Autodesk Inventor part; units mm, degrees
note: some values were not read from the file. Chosen so that the rebuilt part matches the saved one: sketch regions of "Extrusion1".
(part 2 of 3)
  ellipse E482 centre (82.4896, 103.4568) end of major axis (81.6396, 103.4569) minor radius 0.8452 projected
  ellipse E483 centre (90.1098, 108.5077) end of major axis (89.3598, 108.5077) minor radius 0.7458 projected
  ellipse E484 centre (68.5696, 103.4576) end of major axis (66.5696, 103.4577) minor radius 1.9887 projected
  ellipse E485 centre (71.1098, 108.5087) end of major axis (70.3598, 108.5088) minor radius 0.7458 projected
  ellipse E486 centre (95.7978, 108.1793) end of major axis (95.5478, 108.1793) minor radius 0.2486 projected
  ellipse E487 centre (9.5448, 108.1839) end of major axis (9.2948, 108.1839) minor radius 0.2486 projected
  ellipse E488 centre (-152.6552, 108.1925) end of major axis (-152.9052, 108.1925) minor radius 0.2486 projected
  ellipse E489 centre (-102.1004, 103.4667) end of major axis (-102.9504, 103.4667) minor radius 0.8452 projected
  ellipse E490 centre (-112.2604, 103.4672) end of major axis (-113.1104, 103.4673) minor radius 0.8452 projected
  ellipse E491 centre (-104.6402, 108.5181) end of major axis (-105.3902, 108.5181) minor radius 0.7458 projected
  ellipse E492 centre (2.2348, 108.5124) end of major axis (1.4848, 108.5124) minor radius 0.7458 projected
  ellipse E493 centre (-5.3854, 103.4615) end of major axis (-6.2354, 103.4616) minor radius 0.8452 projected
  ellipse E494 centre (-0.3054, 103.4613) end of major axis (-2.3054, 103.4614) minor radius 1.9887 projected
  ellipse E495 centre (-29.1354, 103.4628) end of major axis (-29.9854, 103.4628) minor radius 0.8452 projected
  ellipse E496 centre (-27.8653, 105.9884) end of major axis (-28.6153, 105.9884) minor radius 0.7458 projected
  ellipse E497 centre (-21.5152, 108.5137) end of major axis (-22.2652, 108.5137) minor radius 0.7458 projected
  ellipse E498 centre (-59.6802, 108.1876) end of major axis (-61.0302, 108.1876) minor radius 1.3424 projected
  ellipse E499 centre (-61.112, 109.6114) end of major axis (-61.362, 109.6114) minor radius 0.2486 projected
  ellipse E500 centre (-58.2484, 106.7637) end of major axis (-58.4984, 106.7637) minor radius 0.2486 projected
  ellipse E501 centre (-58.2482, 109.6113) end of major axis (-58.4982, 109.6113) minor radius 0.2486 projected
  ellipse E502 centre (-59.6803, 106.174) end of major axis (-59.9303, 106.174) minor radius 0.2486 projected
  ellipse E503 centre (-57.6552, 108.1875) end of major axis (-57.9052, 108.1875) minor radius 0.2486 projected
  ellipse E504 centre (-59.6801, 110.2011) end of major axis (-59.9301, 110.2011) minor radius 0.2486 projected
  ellipse E505 centre (-50.03, 110.4243) end of major axis (-51.555, 110.4244) minor radius 1.5164 projected
  ellipse E506 centre (-61.7052, 108.1877) end of major axis (-61.9552, 108.1877) minor radius 0.2486 projected
  ellipse E507 centre (-187.7652, 108.5225) end of major axis (-188.5152, 108.5226) minor radius 0.7458 projected
  ellipse E508 centre (-156.1121, 106.7689) end of major axis (-156.3621, 106.7689) minor radius 0.2486 projected
  ellipse E509 centre (-154.6802, 108.1926) end of major axis (-156.0302, 108.1927) minor radius 1.3424 projected
  ellipse E510 centre (-153.2482, 109.6163) end of major axis (-153.4982, 109.6164) minor radius 0.2486 projected
  ellipse E511 centre (-156.112, 109.6165) end of major axis (-156.362, 109.6165) minor radius 0.2486 projected
  ellipse E512 centre (-156.7052, 108.1927) end of major axis (-156.9552, 108.1928) minor radius 0.2486 projected
  ellipse E513 centre (-154.6801, 110.2062) end of major axis (-154.9301, 110.2062) minor radius 0.2486 projected
  ellipse E514 centre (-164.33, 110.4304) end of major axis (-165.855, 110.4305) minor radius 1.5164 projected
  ellipse E515 centre (-190.3054, 103.4714) end of major axis (-192.3054, 103.4715) minor radius 1.9887 projected
  ellipse E516 centre (178.1668, 51.4973) end of major axis (177.9168, 51.4973) minor radius 0.2486 projected
  ellipse E517 centre (132.8568, 51.8278) end of major axis (132.1068, 51.8279) minor radius 0.7458 projected
  ellipse E518 centre (130.3176, 65.6692) end of major axis (128.3176, 65.6693) minor radius 1.9887 projected
  ellipse E519 centre (145.5077, 68.194) end of major axis (144.7577, 68.1941) minor radius 0.7458 projected
  ellipse E520 centre (168.3176, 65.6672) end of major axis (166.3176, 65.6673) minor radius 1.9887 projected
  ellipse E521 centre (149.3176, 65.6682) end of major axis (147.3176, 65.6683) minor radius 1.9887 projected
  ellipse E522 centre (173.3976, 65.6669) end of major axis (172.5476, 65.667) minor radius 0.8452 projected
  ellipse E523 centre (145.5087, 87.0866) end of major axis (144.7587, 87.0866) minor radius 0.7458 projected
  ellipse E524 centre (144.2386, 84.561) end of major axis (143.3886, 84.5611) minor radius 0.8452 projected
  ellipse E525 centre (149.3186, 84.5607) end of major axis (147.3186, 84.5608) minor radius 1.9887 projected
  ellipse E526 centre (168.3186, 84.5597) end of major axis (166.3186, 84.5598) minor radius 1.9887 projected
  ellipse E527 centre (163.2386, 84.56) end of major axis (162.3886, 84.56) minor radius 0.8452 projected
  ellipse E528 centre (139.8182, 77.1285) end of major axis (139.5682, 77.1285) minor radius 0.2486 projected
  ellipse E529 centre (138.3861, 73.6913) end of major axis (138.1361, 73.6913) minor radius 0.2486 projected
  ellipse E530 centre (138.3863, 76.5388) end of major axis (138.1363, 76.5389) minor radius 0.2486 projected
  ellipse E531 centre (141.25, 76.5387) end of major axis (141, 76.5387) minor radius 0.2486 projected
  ellipse E532 centre (139.8181, 75.115) end of major axis (138.4681, 75.115) minor radius 1.3424 projected
  ellipse E533 centre (141.8431, 75.1149) end of major axis (141.5931, 75.1149) minor radius 0.2486 projected
  ellipse E534 centre (135.3986, 84.5615) end of major axis (134.5486, 84.5615) minor radius 0.8452 projected
  ellipse E535 centre (139.818, 73.1014) end of major axis (139.568, 73.1014) minor radius 0.2486 projected
  ellipse E536 centre (126.5087, 87.0876) end of major axis (125.7587, 87.0876) minor radius 0.7458 projected
  ellipse E537 centre (125.2376, 65.6695) end of major axis (124.3876, 65.6695) minor radius 0.8452 projected
  ellipse E538 centre (126.5077, 68.1951) end of major axis (125.7577, 68.1951) minor radius 0.7458 projected
  ellipse E539 centre (63.4886, 84.5653) end of major axis (62.6386, 84.5654) minor radius 0.8452 projected
  ellipse E540 centre (73.6486, 84.5648) end of major axis (72.7986, 84.5648) minor radius 0.8452 projected
  ellipse E541 centre (113.8573, 61.2751) end of major axis (113.1073, 61.2751) minor radius 0.7458 projected
  ellipse E542 centre (118.3177, 68.0563) end of major axis (116.7927, 68.0564) minor radius 1.5164 projected
  ellipse E543 centre (-73.9314, 84.5727) end of major axis (-75.9314, 84.5728) minor radius 1.9887 projected
  ellipse E544 centre (-68.8514, 84.5724) end of major axis (-69.7014, 84.5724) minor radius 0.8452 projected
  ellipse E545 centre (-68.2423, 68.2055) end of major axis (-68.9923, 68.2055) minor radius 0.7458 projected
  ellipse E546 centre (-58.7413, 87.0975) end of major axis (-59.4913, 87.0975) minor radius 0.7458 projected
  ellipse E547 centre (-61.8922, 70.7307) end of major axis (-62.6422, 70.7308) minor radius 0.7458 projected
  ellipse E548 centre (-50.5124, 65.6789) end of major axis (-51.3624, 65.6789) minor radius 0.8452 projected
  ellipse E549 centre (-69.5124, 65.6799) end of major axis (-70.3624, 65.6799) minor radius 0.8452 projected
  ellipse E550 centre (-49.2423, 68.2044) end of major axis (-49.9923, 68.2045) minor radius 0.7458 projected
  ellipse E551 centre (-21.3524, 65.6773) end of major axis (-22.2024, 65.6774) minor radius 0.8452 projected
  ellipse E552 centre (-26.4324, 65.6776) end of major axis (-28.4324, 65.6777) minor radius 1.9887 projected
  ellipse E553 centre (-26.4319, 75.7264) end of major axis (-27.7819, 75.7265) minor radius 1.3424 projected
  ellipse E554 centre (-27.8639, 74.3027) end of major axis (-28.1139, 74.3027) minor radius 0.2486 projected
  ellipse E555 centre (-35.9314, 84.5706) end of major axis (-37.9314, 84.5707) minor radius 1.9887 projected
  ellipse E556 centre (-20.7413, 87.0954) end of major axis (-21.4913, 87.0955) minor radius 0.7458 projected
  ellipse E557 centre (-40.3524, 65.6783) end of major axis (-41.2024, 65.6784) minor radius 0.8452 projected
  ellipse E558 centre (-39.7413, 87.0965) end of major axis (-40.4913, 87.0965) minor radius 0.7458 projected
  ellipse E559 centre (-42.8922, 70.7297) end of major axis (-43.6422, 70.7298) minor radius 0.7458 projected
  ellipse E560 centre (-45.4324, 65.6786) end of major axis (-47.4324, 65.6787) minor radius 1.9887 projected
  ellipse E561 centre (13.9436, 84.568) end of major axis (11.9436, 84.5681) minor radius 1.9887 projected
  ellipse E562 centre (10.1337, 87.0938) end of major axis (9.3837, 87.0938) minor radius 0.7458 projected
  ellipse E563 centre (2.0431, 76.3752) end of major axis (0.0431, 76.3753) minor radius 1.9887 projected
  ellipse E564 centre (-16.9314, 84.5696) end of major axis (-18.9314, 84.5697) minor radius 1.9887 projected
  ellipse E565 centre (-2.3524, 65.6763) end of major axis (-3.2024, 65.6763) minor radius 0.8452 projected
  ellipse E566 centre (31.9998, 71.8214) end of major axis (31.7498, 71.8214) minor radius 0.2486 projected
  ellipse E567 centre (25.8431, 76.3739) end of major axis (23.8431, 76.374) minor radius 1.9887 projected
  ellipse E568 centre (31.9996, 68.9738) end of major axis (31.7496, 68.9738) minor radius 0.2486 projected
  ellipse E569 centre (30.5678, 70.3977) end of major axis (29.2178, 70.3977) minor radius 1.3424 projected
  ellipse E570 centre (28.5428, 70.3978) end of major axis (28.2928, 70.3978) minor radius 0.2486 projected
  ellipse E571 centre (18.6926, 65.6752) end of major axis (16.6926, 65.6753) minor radius 1.9887 projected
  ellipse E572 centre (21.2328, 70.7263) end of major axis (20.4828, 70.7263) minor radius 0.7458 projected
  ellipse E573 centre (-0.1432, 51.8349) end of major axis (-0.8932, 51.835) minor radius 0.7458 projected
  ellipse E574 centre (-57.1432, 51.838) end of major axis (-57.8932, 51.838) minor radius 0.7458 projected
  ellipse E575 centre (-76.1432, 51.839) end of major axis (-76.8932, 51.839) minor radius 0.7458 projected
  ellipse E576 centre (23.6068, 51.8336) end of major axis (22.8568, 51.8337) minor radius 0.7458 projected
  ellipse E577 centre (32.5928, 70.3976) end of major axis (32.3428, 70.3976) minor radius 0.2486 projected
  ellipse E578 centre (-109.907, 74.4681) end of major axis (-110.157, 74.4681) minor radius 0.2486 projected
  ellipse E579 centre (-102.4324, 65.6816) end of major axis (-104.4324, 65.6817) minor radius 1.9887 projected
  ellipse E580 centre (-78.3524, 65.6804) end of major axis (-79.2024, 65.6804) minor radius 0.8452 projected
  ellipse E581 centre (-88.5124, 65.6809) end of major axis (-89.3624, 65.6809) minor radius 0.8452 projected
  ellipse E582 centre (-87.2423, 68.2065) end of major axis (-87.9923, 68.2065) minor radius 0.7458 projected
  ellipse E583 centre (-96.7413, 87.0995) end of major axis (-97.4913, 87.0995) minor radius 0.7458 projected
  ellipse E584 centre (-110.5002, 73.0443) end of major axis (-110.7502, 73.0443) minor radius 0.2486 projected
  ellipse E585 centre (-191.7413, 87.1046) end of major axis (-192.4913, 87.1046) minor radius 0.7458 projected
  ellipse E586 centre (-187.9314, 84.5787) end of major axis (-189.9314, 84.5788) minor radius 1.9887 projected
  ellipse E587 centre (-174.0114, 84.578) end of major axis (-174.8614, 84.578) minor radius 0.8452 projected
  ellipse E588 centre (-172.7413, 87.1036) end of major axis (-173.4913, 87.1036) minor radius 0.7458 projected
  ellipse E589 centre (-153.7413, 87.1025) end of major axis (-154.4913, 87.1026) minor radius 0.7458 projected
  ellipse E590 centre (-163.8514, 84.5775) end of major axis (-164.7014, 84.5775) minor radius 0.8452 projected
  ellipse E591 centre (-113.3638, 75.892) end of major axis (-113.6138, 75.8921) minor radius 0.2486 projected
  ellipse E592 centre (-111.932, 74.4682) end of major axis (-113.282, 74.4682) minor radius 1.3424 projected
  ellipse E593 centre (-110.5, 75.8919) end of major axis (-110.75, 75.8919) minor radius 0.2486 projected
  ellipse E594 centre (-113.957, 74.4683) end of major axis (-114.207, 74.4683) minor radius 0.2486 projected
  ellipse E595 centre (-117.0114, 84.575) end of major axis (-117.8614, 84.575) minor radius 0.8452 projected
  ellipse E596 centre (-115.7413, 87.1005) end of major axis (-116.4913, 87.1006) minor radius 0.7458 projected
  ellipse E597 centre (-130.9314, 84.5757) end of major axis (-132.9314, 84.5758) minor radius 1.9887 projected
  ellipse E598 centre (-149.9314, 84.5767) end of major axis (-151.9314, 84.5768) minor radius 1.9887 projected
  ellipse E599 centre (-182.2423, 68.2115) end of major axis (-182.9923, 68.2116) minor radius 0.7458 projected
  ellipse E600 centre (-183.5124, 65.686) end of major axis (-184.3624, 65.686) minor radius 0.8452 projected
  ellipse E601 centre (-178.4324, 65.6857) end of major axis (-180.4324, 65.6858) minor radius 1.9887 projected
  ellipse E602 centre (-163.2423, 68.2105) end of major axis (-163.9923, 68.2106) minor radius 0.7458 projected
  ellipse E603 centre (-137.8922, 70.7348) end of major axis (-138.6422, 70.7348) minor radius 0.7458 projected
  ellipse E604 centre (-144.2423, 68.2095) end of major axis (-144.9923, 68.2095) minor radius 0.7458 projected
  ellipse E605 centre (-140.4324, 65.6837) end of major axis (-142.4324, 65.6838) minor radius 1.9887 projected
  ellipse E606 centre (-126.5124, 65.6829) end of major axis (-127.3624, 65.683) minor radius 0.8452 projected
  ellipse E607 centre (-135.3524, 65.6834) end of major axis (-136.2024, 65.6834) minor radius 0.8452 projected
  ellipse E608 centre (-111.9321, 72.4546) end of major axis (-112.1821, 72.4546) minor radius 0.2486 projected
  ellipse E609 centre (-118.8922, 70.7338) end of major axis (-119.6422, 70.7338) minor radius 0.7458 projected
  ellipse E610 centre (-192.3524, 65.6864) end of major axis (-193.2024, 65.6865) minor radius 0.8452 projected
  ellipse E611 centre (-133.1432, 51.842) end of major axis (-133.8932, 51.8421) minor radius 0.7458 projected
  ellipse E612 centre (-171.1432, 51.844) end of major axis (-171.8932, 51.8441) minor radius 0.7458 projected
  ellipse E613 centre (107.5092, 96.5349) end of major axis (106.7592, 96.5349) minor radius 0.7458 projected
  ellipse E614 centre (-14.3912, 89.6207) end of major axis (-15.1412, 89.6208) minor radius 0.7458 projected
  ellipse E615 centre (25.8439, 91.5277) end of major axis (24.3189, 91.5278) minor radius 1.5164 projected
  ellipse E616 centre (132.8588, 89.6129) end of major axis (132.1088, 89.6129) minor radius 0.7458 projected
  ellipse E617 centre (116.3991, 94.0088) end of major axis (115.5491, 94.0088) minor radius 0.8452 projected
  ellipse E618 centre (-90.3912, 89.6248) end of major axis (-91.1412, 89.6248) minor radius 0.7458 projected
  ellipse E619 centre (-71.3912, 89.6238) end of major axis (-72.1412, 89.6238) minor radius 0.7458 projected
  ellipse E620 centre (-164.3309, 95.2766) end of major axis (-166.3309, 95.2767) minor radius 1.9887 projected
  ellipse E621 centre (-166.3912, 89.6289) end of major axis (-167.1412, 89.6289) minor radius 0.7458 projected
  ellipse E622 centre (181.6238, 52.9209) end of major axis (181.3738, 52.9209) minor radius 0.2486 projected
  ellipse E623 centre (178.76, 52.921) end of major axis (178.51, 52.921) minor radius 0.2486 projected
  ellipse E624 centre (180.1919, 53.5107) end of major axis (179.9419, 53.5107) minor radius 0.2486 projected
  ellipse E625 centre (178.757, -3.7566) end of major axis (178.507, -3.7566) minor radius 0.2486 projected
  ellipse E626 centre (73.8545, 8.9399) end of major axis (73.4545, 8.94) minor radius 0.3977 projected
  ellipse E627 centre (81.4745, 8.9395) end of major axis (81.0745, 8.9396) minor radius 0.3977 projected
  ellipse E628 centre (125.2366, 46.777) end of major axis (124.3866, 46.777) minor radius 0.8452 projected
  ellipse E629 centre (126.5057, 30.41) end of major axis (125.7557, 30.41) minor radius 0.7458 projected
  ellipse E630 centre (135.3966, 46.7764) end of major axis (134.5466, 46.7765) minor radius 0.8452 projected
  ellipse E631 centre (137.791, 37.33) end of major axis (137.541, 37.33) minor radius 0.2486 projected
  ellipse E632 centre (154.3966, 46.7754) end of major axis (153.5466, 46.7754) minor radius 0.8452 projected
  ellipse E633 centre (141.841, 37.3298) end of major axis (141.591, 37.3298) minor radius 0.2486 projected
  ellipse E634 centre (138.3841, 35.9062) end of major axis (138.1341, 35.9062) minor radius 0.2486 projected
  ellipse E635 centre (139.816, 37.3299) end of major axis (138.466, 37.33) minor radius 1.3424 projected
  ellipse E636 centre (141.248, 38.7536) end of major axis (140.998, 38.7536) minor radius 0.2486 projected
  ellipse E637 centre (151.8558, 32.9343) end of major axis (151.1058, 32.9343) minor radius 0.7458 projected
  ellipse E638 centre (139.8159, 35.3164) end of major axis (139.5659, 35.3164) minor radius 0.2486 projected
  ellipse E639 centre (149.3155, 27.8831) end of major axis (147.3155, 27.8832) minor radius 1.9887 projected
  ellipse E640 centre (125.2355, 27.8844) end of major axis (124.3855, 27.8845) minor radius 0.8452 projected
  ellipse E641 centre (135.3955, 27.8839) end of major axis (134.5455, 27.8839) minor radius 0.8452 projected
  ellipse E642 centre (106.2355, 27.8854) end of major axis (105.3855, 27.8855) minor radius 0.8452 projected
  ellipse E643 centre (168.3155, 27.8821) end of major axis (166.3155, 27.8822) minor radius 1.9887 projected
  ellipse E644 centre (173.3966, 46.7744) end of major axis (172.5466, 46.7744) minor radius 0.8452 projected
  ellipse E645 centre (103.0764, 44.3917) end of major axis (101.0764, 44.3918) minor radius 1.9887 projected
  ellipse E646 centre (76.041, 37.3333) end of major axis (75.791, 37.3333) minor radius 0.2486 projected
  ellipse E647 centre (44.4866, 46.7813) end of major axis (43.6366, 46.7813) minor radius 0.8452 projected
  ellipse E648 centre (45.7557, 30.4143) end of major axis (45.0057, 30.4143) minor radius 0.7458 projected
  ellipse E649 centre (71.3145, 8.9401) end of major axis (70.9145, 8.9401) minor radius 0.3977 projected
  ellipse E650 centre (66.2345, 8.9403) end of major axis (65.8345, 8.9404) minor radius 0.3977 projected
  ellipse E651 centre (56.0745, 8.9409) end of major axis (55.6745, 8.9409) minor radius 0.3977 projected
  ellipse E652 centre (52.351, -1.1614) end of major axis (51.851, -1.1614) minor radius 0.4972 projected
  ellipse E653 centre (-9.6457, 4.6041) end of major axis (-10.3957, 4.6041) minor radius 0.7458 projected
  ellipse E654 centre (9.9939, -3.3318) end of major axis (9.5939, -3.3318) minor radius 0.3977 projected
  ellipse E655 centre (36.257, -3.749) end of major axis (36.007, -3.749) minor radius 0.2486 projected
  ellipse E656 centre (7.1662, 39.6986) end of major axis (6.9162, 39.6986) minor radius 0.2486 projected
  ellipse E657 centre (28.3558, 32.9409) end of major axis (27.6058, 32.9409) minor radius 0.7458 projected
  ellipse E658 centre (26.1466, 46.7822) end of major axis (25.2966, 46.7823) minor radius 0.8452 projected
  ellipse E659 centre (126.5067, 49.3025) end of major axis (125.7567, 49.3026) minor radius 0.7458 projected
  ellipse E660 centre (-72.9958, 2.0818) end of major axis (-73.7458, 2.0819) minor radius 0.7458 projected
  ellipse E661 centre (-69.1838, 40.1103) end of major axis (-69.4338, 40.1103) minor radius 0.2486 projected
  ellipse E662 centre (-69.184, 36.0832) end of major axis (-69.434, 36.0832) minor radius 0.2486 projected
  ellipse E663 centre (-67.7521, 36.6729) end of major axis (-68.0021, 36.6729) minor radius 0.2486 projected
  ellipse E664 centre (-69.1839, 38.0968) end of major axis (-70.5339, 38.0968) minor radius 1.3424 projected
  ellipse E665 centre (-50.1845, 27.8938) end of major axis (-52.1845, 27.8939) minor radius 1.9887 projected
  ellipse E666 centre (-36.266, -0.4458) end of major axis (-37.116, -0.4457) minor radius 0.8452 projected
  ellipse E667 centre (-34.9958, 2.0798) end of major axis (-35.7458, 2.0798) minor radius 0.7458 projected
  ellipse E668 centre (-66.6457, 4.6071) end of major axis (-67.3957, 4.6072) minor radius 0.7458 projected
  ellipse E669 centre (-69.186, -0.444) end of major axis (-71.186, -0.4439) minor radius 1.9887 projected
  ellipse E670 centre (-54.6034, 46.7866) end of major axis (-55.4534, 46.7866) minor radius 0.8452 projected
  ellipse E671 centre (-40.6834, 46.7858) end of major axis (-42.6834, 46.7859) minor radius 1.9887 projected
  ellipse E672 centre (-45.7634, 46.7861) end of major axis (-46.6134, 46.7861) minor radius 0.8452 projected
  ellipse E673 centre (-35.6034, 46.7855) end of major axis (-36.4534, 46.7856) minor radius 0.8452 projected
  ellipse E674 centre (-64.7634, 46.7871) end of major axis (-65.6134, 46.7871) minor radius 0.8452 projected
  ellipse E675 centre (-26.106, -0.4463) end of major axis (-26.956, -0.4463) minor radius 0.8452 projected
  ellipse E676 centre (-26.1045, 27.8925) end of major axis (-26.9545, 27.8925) minor radius 0.8452 projected
  ellipse E677 centre (17.2567, 49.3084) end of major axis (16.5067, 49.3084) minor radius 0.7458 projected
  ellipse E678 centre (15.9866, 46.7828) end of major axis (15.1366, 46.7828) minor radius 0.8452 projected
  ellipse E679 centre (10.6231, 41.1222) end of major axis (10.3731, 41.1222) minor radius 0.2486 projected
  ellipse E680 centre (11.8955, 27.8905) end of major axis (11.0455, 27.8905) minor radius 0.8452 projected
  ellipse E681 centre (7.7592, 38.2747) end of major axis (7.5092, 38.2747) minor radius 0.2486 projected
  ellipse E682 centre (6.8155, 27.8907) end of major axis (4.8155, 27.8909) minor radius 1.9887 projected
  ellipse E683 centre (-16.6034, 46.7845) end of major axis (-17.4534, 46.7846) minor radius 0.8452 projected
  ellipse E684 centre (-7.1045, 27.8915) end of major axis (-7.9545, 27.8915) minor radius 0.8452 projected
  ellipse E685 centre (-17.266, -0.4468) end of major axis (-18.116, -0.4467) minor radius 0.8452 projected
  ellipse E686 centre (-15.9958, 2.0788) end of major axis (-16.7458, 2.0788) minor radius 0.7458 projected
  ellipse E687 centre (64.7567, 49.3058) end of major axis (64.0067, 49.3059) minor radius 0.7458 projected
  ellipse E688 centre (64.7557, 30.4133) end of major axis (64.0057, 30.4133) minor radius 0.7458 projected
  ellipse E689 centre (52.3513, 3.8898) end of major axis (51.8513, 3.8899) minor radius 0.4972 projected
  ellipse E690 centre (61.1545, 8.9406) end of major axis (60.7545, 8.9406) minor radius 0.3977 projected
  ellipse E691 centre (44.9851, 0.2062) end of major axis (44.6101, 0.2062) minor radius 0.3729 projected
  ellipse E692 centre (-148.9943, 30.4247) end of major axis (-149.7443, 30.4247) minor radius 0.7458 projected
  ellipse E693 centre (-129.9943, 30.4237) end of major axis (-130.7443, 30.4237) minor radius 0.7458 projected
  ellipse E694 centre (-140.1045, 27.8986) end of major axis (-140.9545, 27.8986) minor radius 0.8452 projected
  ellipse E695 centre (-131.2645, 27.8981) end of major axis (-132.1145, 27.8982) minor radius 0.8452 projected
  ellipse E696 centre (-95.1457, 4.6087) end of major axis (-95.8957, 4.6087) minor radius 0.7458 projected
  ellipse E697 centre (-112.2645, 27.8971) end of major axis (-113.1145, 27.8971) minor radius 0.8452 projected
  ellipse E698 centre (-107.1845, 27.8968) end of major axis (-109.1845, 27.8969) minor radius 1.9887 projected
  ellipse E699 centre (-92.606, -0.4427) end of major axis (-93.456, -0.4427) minor radius 0.8452 projected
  ellipse E700 centre (-102.766, -0.4422) end of major axis (-103.616, -0.4422) minor radius 0.8452 projected
  ellipse E701 centre (-97.686, -0.4425) end of major axis (-99.686, -0.4424) minor radius 1.9887 projected
  ellipse E702 centre (-139.4958, 2.0854) end of major axis (-140.2458, 2.0854) minor radius 0.7458 projected
  ellipse E703 centre (-149.6034, 46.7916) end of major axis (-150.4534, 46.7917) minor radius 0.8452 projected
  ellipse E704 centre (-92.6034, 46.7886) end of major axis (-93.4534, 46.7886) minor radius 0.8452 projected
  ellipse E705 centre (-139.4933, 49.3167) end of major axis (-140.2433, 49.3168) minor radius 0.7458 projected
  ellipse E706 centre (-82.4933, 49.3137) end of major axis (-83.2433, 49.3137) minor radius 0.7458 projected
  ellipse E707 centre (-83.4361, -3.1528) end of major axis (-83.6861, -3.1528) minor radius 0.2486 projected
  ellipse E708 centre (-168.9361, -3.1483) end of major axis (-169.1861, -3.1482) minor radius 0.2486 projected
  ellipse E709 centre (-169.2645, 27.9001) end of major axis (-170.1145, 27.9002) minor radius 0.8452 projected
  ellipse E710 centre (-159.7634, 46.7922) end of major axis (-160.6134, 46.7922) minor radius 0.8452 projected
  ellipse E711 centre (-159.1045, 27.8996) end of major axis (-159.9545, 27.8996) minor radius 0.8452 projected
  ellipse E712 centre (-152.1457, 4.6117) end of major axis (-152.8957, 4.6117) minor radius 0.7458 projected
  ellipse E713 centre (-187.6034, 46.7937) end of major axis (-188.4534, 46.7937) minor radius 0.8452 projected
  ellipse E714 centre (-170.368, -3.7379) end of major axis (-170.618, -3.7379) minor radius 0.2486 projected
  ellipse E715 centre (-180.6457, 4.6132) end of major axis (-181.3957, 4.6133) minor radius 0.7458 projected
  ellipse E716 centre (-177.4933, 49.3188) end of major axis (-178.2433, 49.3188) minor radius 0.7458 projected
  ellipse E717 centre (178.7598, 50.0734) end of major axis (178.5098, 50.0735) minor radius 0.2486 projected
  ellipse E718 centre (181.6207, -3.7567) end of major axis (181.3707, -3.7567) minor radius 0.2486 projected
  ellipse E719 centre (180.1889, -3.1669) end of major axis (179.9389, -3.1669) minor radius 0.2486 projected
  ellipse E720 centre (181.6236, 50.0733) end of major axis (181.3736, 50.0733) minor radius 0.2486 projected
  ellipse E721 centre (180.1918, 51.4972) end of major axis (178.8418, 51.4972) minor radius 1.3424 projected
  ellipse E722 centre (180.1917, 49.4836) end of major axis (179.9417, 49.4836) minor radius 0.2486 projected
  ellipse E723 centre (-211.5152, 108.5238) end of major axis (-212.2652, 108.5238) minor radius 0.7458 projected
  ellipse E724 centre (-202.1811, 91.6642) end of major axis (-203.5311, 91.6643) minor radius 1.3424 projected
  ellipse E725 centre (-204.2061, 91.6643) end of major axis (-204.4561, 91.6643) minor radius 0.2486 projected
  ellipse E726 centre (-201.2423, 68.2126) end of major axis (-201.9923, 68.2126) minor radius 0.7458 projected
  ellipse E727 centre (-209.1432, 51.8461) end of major axis (-209.8932, 51.8461) minor radius 0.7458 projected
  ellipse E728 centre (-205.9958, 2.0889) end of major axis (-206.7458, 2.089) minor radius 0.7458 projected
  ellipse E729 centre (180.1887, -7.194) end of major axis (179.9387, -7.194) minor radius 0.2486 projected
  ellipse E730 centre (178.7568, -6.6042) end of major axis (178.5068, -6.6041) minor radius 0.2486 projected
  ellipse E731 centre (178.1638, -5.1803) end of major axis (177.9138, -5.1803) minor radius 0.2486 projected
  ellipse E732 centre (181.6206, -6.6043) end of major axis (181.3706, -6.6043) minor radius 0.2486 projected
  ellipse E733 centre (180.1888, -5.1804) end of major axis (178.8388, -5.1804) minor radius 1.3424 projected
  ellipse E734 centre (182.2198, 108.1746) end of major axis (181.9698, 108.1747) minor radius 0.2486 projected
  ellipse E735 centre (182.2168, 51.497) end of major axis (181.9668, 51.4971) minor radius 0.2486 projected
  ellipse E736 centre (182.2138, -5.1806) end of major axis (181.9638, -5.1805) minor radius 0.2486 projected
  ellipse E737 centre (-252.0552, 108.1978) end of major axis (-253.4052, 108.1979) minor radius 1.3424 projected
  ellipse E738 centre (-250.6234, 106.774) end of major axis (-250.8734, 106.774) minor radius 0.2486 projected
  ellipse E739 centre (-253.4871, 106.7741) end of major axis (-253.7371, 106.7741) minor radius 0.2486 projected
  ellipse E740 centre (-250.6232, 109.6215) end of major axis (-250.8732, 109.6216) minor radius 0.2486 projected
  ellipse E741 centre (-253.487, 109.6217) end of major axis (-253.737, 109.6217) minor radius 0.2486 projected
  ellipse E742 centre (-252.0553, 106.1843) end of major axis (-252.3053, 106.1843) minor radius 0.2486 projected
  ellipse E743 centre (-250.6262, 52.9439) end of major axis (-250.8762, 52.944) minor radius 0.2486 projected
  ellipse E744 centre (-252.0582, 51.5202) end of major axis (-253.4082, 51.5203) minor radius 1.3424 projected
  ellipse E745 centre (-250.6264, 50.0964) end of major axis (-250.8764, 50.0964) minor radius 0.2486 projected
  ellipse E746 centre (-253.4902, 50.0965) end of major axis (-253.7402, 50.0965) minor radius 0.2486 projected
  ellipse E747 centre (-253.49, 52.9441) end of major axis (-253.74, 52.9441) minor radius 0.2486 projected
  ellipse E748 centre (-252.0581, 53.5338) end of major axis (-252.3081, 53.5338) minor radius 0.2486 projected
  ellipse E749 centre (-253.4932, -6.5811) end of major axis (-253.7432, -6.5811) minor radius 0.2486 projected
  ellipse E750 centre (-252.0612, -5.1574) end of major axis (-253.4112, -5.1573) minor radius 1.3424 projected
  ellipse E751 centre (-250.6294, -6.5812) end of major axis (-250.8794, -6.5812) minor radius 0.2486 projected
  ellipse E752 centre (-253.493, -3.7335) end of major axis (-253.743, -3.7335) minor radius 0.2486 projected
  ellipse E753 centre (-250.6293, -3.7337) end of major axis (-250.8793, -3.7336) minor radius 0.2486 projected
  ellipse E754 centre (-252.0611, -3.1438) end of major axis (-252.3111, -3.1438) minor radius 0.2486 projected
  ellipse E755 centre (-252.0583, 49.5067) end of major axis (-252.3083, 49.5067) minor radius 0.2486 projected
  ellipse E756 centre (-240.5134, 46.7965) end of major axis (-241.3634, 46.7965) minor radius 0.8452 projected
  ellipse E757 centre (-239.2433, 49.322) end of major axis (-239.9933, 49.3221) minor radius 0.7458 projected
  ellipse E758 centre (-250.0332, 51.5201) end of major axis (-250.2832, 51.5201) minor radius 0.2486 projected
  ellipse E759 centre (-242.5841, 34.8645) end of major axis (-244.1091, 34.8645) minor radius 1.5164 projected
  ellipse E760 centre (-242.8854, 103.4742) end of major axis (-243.7354, 103.4743) minor radius 0.8452 projected
  ellipse E761 centre (-240.2071, 72.6494) end of major axis (-241.7321, 72.6495) minor radius 1.5164 projected
  ellipse E762 centre (-242.5849, 19.7107) end of major axis (-244.5849, 19.7108) minor radius 1.9887 projected
  ellipse E763 centre (-250.0362, -5.1575) end of major axis (-250.2862, -5.1575) minor radius 0.2486 projected
  ellipse E764 centre (-240.186, -0.4349) end of major axis (-242.186, -0.4348) minor radius 1.9887 projected
  ellipse E765 centre (-243.9958, 2.091) end of major axis (-244.7458, 2.091) minor radius 0.7458 projected
  ellipse E766 centre (-245.266, -0.4346) end of major axis (-246.116, -0.4346) minor radius 0.8452 projected
  ellipse E767 centre (-250.0302, 108.1977) end of major axis (-250.2802, 108.1977) minor radius 0.2486 projected
  ellipse E768 centre (-224.9906, 41.1347) end of major axis (-225.2406, 41.1348) minor radius 0.2486 projected
  ellipse E769 centre (-223.5588, 39.7109) end of major axis (-224.9088, 39.7109) minor radius 1.3424 projected
  ellipse E770 centre (-222.127, 38.287) end of major axis (-222.377, 38.287) minor radius 0.2486 projected
  ellipse E771 centre (-224.9908, 38.2872) end of major axis (-225.2408, 38.2872) minor radius 0.2486 projected
  ellipse E772 centre (-222.1269, 41.1346) end of major axis (-222.3769, 41.1346) minor radius 0.2486 projected
  ellipse E773 centre (-225.5838, 39.711) end of major axis (-225.8338, 39.711) minor radius 0.2486 projected
  ellipse E774 centre (-223.5589, 37.6973) end of major axis (-223.8089, 37.6973) minor radius 0.2486 projected
  ellipse E775 centre (-235.7645, 27.9037) end of major axis (-236.6145, 27.9037) minor radius 0.8452 projected
  ellipse E776 centre (-234.4943, 30.4293) end of major axis (-235.2443, 30.4293) minor radius 0.7458 projected
  ellipse E777 centre (-228.1442, 32.9546) end of major axis (-228.8942, 32.9546) minor radius 0.7458 projected
  ellipse E778 centre (-230.6845, 27.9034) end of major axis (-232.6845, 27.9035) minor radius 1.9887 projected
  ellipse E779 centre (-225.6045, 27.9032) end of major axis (-226.4545, 27.9032) minor radius 0.8452 projected
  ellipse E780 centre (-235.106, -0.4351) end of major axis (-235.956, -0.4351) minor radius 0.8452 projected
  ellipse E781 centre (-226.266, -0.4356) end of major axis (-227.116, -0.4356) minor radius 0.8452 projected
  ellipse E782 centre (-224.9958, 2.09) end of major axis (-225.7458, 2.09) minor radius 0.7458 projected
  ellipse E783 centre (-221.186, -0.4359) end of major axis (-223.186, -0.4358) minor radius 1.9887 projected
  ellipse E784 centre (-235.4334, 46.7962) end of major axis (-237.4334, 46.7963) minor radius 1.9887 projected
  ellipse E785 centre (-237.6457, 4.6163) end of major axis (-238.3957, 4.6163) minor radius 0.7458 projected
  ellipse E786 centre (-230.3534, 46.7959) end of major axis (-231.2034, 46.796) minor radius 0.8452 projected
  ellipse E787 centre (-228.6364, 84.5809) end of major axis (-229.4864, 84.581) minor radius 0.8452 projected
  ellipse E788 centre (-235.4569, 76.3879) end of major axis (-237.4569, 76.388) minor radius 1.9887 projected
  ellipse E789 centre (-233.3874, 65.6886) end of major axis (-234.2374, 65.6887) minor radius 0.8452 projected
  ellipse E790 centre (-232.1173, 68.2142) end of major axis (-232.8673, 68.2142) minor radius 0.7458 projected
  ellipse E791 centre (-228.3074, 65.6884) end of major axis (-230.3074, 65.6885) minor radius 1.9887 projected
  ellipse E792 centre (-225.7672, 70.7395) end of major axis (-226.5172, 70.7395) minor radius 0.7458 projected
  ellipse E793 centre (-240.2079, 57.4956) end of major axis (-242.2079, 57.4957) minor radius 1.9887 projected
  ellipse E794 centre (-232.8932, 51.8473) end of major axis (-233.6432, 51.8474) minor radius 0.7458 projected
  ellipse E795 centre (-235.4561, 91.5417) end of major axis (-236.9811, 91.5418) minor radius 1.5164 projected
  ellipse E796 centre (-227.3663, 87.1065) end of major axis (-228.1163, 87.1065) minor radius 0.7458 projected
  ellipse E797 centre (-232.7254, 103.4737) end of major axis (-233.5754, 103.4737) minor radius 0.8452 projected
  ellipse E798 centre (-237.8054, 103.4739) end of major axis (-239.8054, 103.474) minor radius 1.9887 projected
  ellipse E799 centre (-241.6153, 105.9998) end of major axis (-242.3653, 105.9998) minor radius 0.7458 projected
  ellipse E800 centre (-235.2652, 108.5251) end of major axis (-236.0152, 108.5251) minor radius 0.7458 projected
  ellipse E801 centre (-221.5338, 39.7108) end of major axis (-221.7838, 39.7108) minor radius 0.2486 projected
  ellipse E802 centre (-223.5587, 41.7244) end of major axis (-223.8087, 41.7244) minor radius 0.2486 projected
  ellipse E803 centre (-221.0162, 89.6318) end of major axis (-221.7662, 89.6318) minor radius 0.7458 projected
  ellipse E804 centre (-223.5564, 84.5806) end of major axis (-225.5564, 84.5807) minor radius 1.9887 projected
  ellipse E805 centre (-223.2274, 65.6881) end of major axis (-224.0774, 65.6881) minor radius 0.8452 projected
  ellipse E806 centre (-252.0613, -7.1709) end of major axis (-252.3113, -7.1709) minor radius 0.2486 projected
  ellipse E807 centre (-252.0551, 110.2114) end of major axis (-252.3051, 110.2114) minor radius 0.2486 projected
  ellipse E808 centre (97.8229, 110.1927) end of major axis (97.5729, 110.1927) minor radius 0.2486 projected
  ellipse E809 centre (11.5699, 110.1973) end of major axis (11.3199, 110.1973) minor radius 0.2486 projected
  ellipse E810 centre (180.1949, 110.1883) end of major axis (179.9449, 110.1883) minor radius 0.2486 projected
  ellipse E811 centre (-254.0862, -5.1573) end of major axis (-254.3362, -5.1572) minor radius 0.2486 projected
  ellipse E812 centre (-254.0832, 51.5203) end of major axis (-254.3332, 51.5204) minor radius 0.2486 projected
  ellipse E813 centre (-254.0802, 108.1979) end of major axis (-254.3302, 108.198) minor radius 0.2486 projected
  line L10 (175.7291, 10.7288) -> (169.2949, -6.8459) projected
  line L11 (169.2949, -6.8459) -> (166.7949, -6.8458) projected
  line L12 (166.7949, -6.8458) -> (173.2291, 10.7289) projected
  line L13 (173.2291, 10.7289) -> (175.7291, 10.7288) projected
  line L14 (165.7291, 10.7293) -> (159.2949, -6.8454) projected
  line L15 (159.2949, -6.8454) -> (156.7949, -6.8452) projected
  line L16 (156.7949, -6.8452) -> (163.2291, 10.7294) projected
  line L17 (163.2291, 10.7294) -> (165.7291, 10.7293) projected
  line L18 (155.7291, 10.7298) -> (149.2949, -6.8448) projected
  line L19 (149.2949, -6.8448) -> (146.7949, -6.8447) projected
  line L20 (146.7949, -6.8447) -> (153.2291, 10.73) projected
  line L21 (153.2291, 10.73) -> (155.7291, 10.7298) projected
  line L22 (145.7291, 10.7304) -> (139.2949, -6.8443) projected
  line L23 (139.2949, -6.8443) -> (136.7949, -6.8442) projected
  line L24 (136.7949, -6.8442) -> (143.2291, 10.7305) projected
  line L25 (143.2291, 10.7305) -> (145.7291, 10.7304) projected
  line L26 (135.7291, 10.7309) -> (129.2949, -6.8438) projected
  line L27 (129.2949, -6.8438) -> (126.7949, -6.8436) projected
  line L28 (126.7949, -6.8436) -> (133.2291, 10.731) projected
  line L29 (133.2291, 10.731) -> (135.7291, 10.7309) projected
  line L30 (125.7291, 10.7314) -> (119.2949, -6.8432) projected
  line L31 (119.2949, -6.8432) -> (116.7949, -6.8431) projected
  line L32 (116.7949, -6.8431) -> (123.2291, 10.7316) projected
  line L33 (123.2291, 10.7316) -> (125.7291, 10.7314) projected
  line L34 (115.7291, 10.732) -> (109.2949, -6.8427) projected
  line L35 (109.2949, -6.8427) -> (106.7949, -6.8426) projected
  line L36 (106.7949, -6.8426) -> (113.2291, 10.7321) projected
  line L37 (113.2291, 10.7321) -> (115.7291, 10.732) projected
  line L38 (105.7291, 10.7325) -> (99.2949, -6.8422) projected
  line L39 (99.2949, -6.8422) -> (96.7949, -6.842) projected
  line L40 (96.7949, -6.842) -> (103.2291, 10.7326) projected
  line L41 (103.2291, 10.7326) -> (105.7291, 10.7325) projected
  line L42 (98.2293, 10.7329) -> (100.7293, 10.7328) projected
  line L43 (100.7293, 10.7328) -> (95.4539, -3.677) projected
  line L44 (95.4539, -3.677) -> (95.4542, 3.1529) projected
  line L45 (95.4542, 3.1529) -> (98.2293, 10.7329) projected
  line L46 (105.3349, 16.4848) -> (107.8349, 16.4847) projected
  line L47 (107.8349, 16.4847) -> (106.4025, 12.572) projected
  line L48 (106.4025, 12.572) -> (103.9025, 12.5721) projected
  line L49 (103.9025, 12.5721) -> (105.3349, 16.4848) projected
  line L50 (115.3349, 16.4843) -> (117.8349, 16.4841) projected
  line L51 (117.8349, 16.4841) -> (116.4025, 12.5715) projected
  line L52 (116.4025, 12.5715) -> (113.9025, 12.5716) projected
  line L53 (113.9025, 12.5716) -> (115.3349, 16.4843) projected
  line L54 (125.3349, 16.4837) -> (127.8349, 16.4836) projected
  line L55 (127.8349, 16.4836) -> (126.4025, 12.5709) projected
  line L56 (126.4025, 12.5709) -> (123.9025, 12.5711) projected
  line L57 (123.9025, 12.5711) -> (125.3349, 16.4837) projected
  line L58 (135.3349, 16.4832) -> (137.8349, 16.4831) projected
  line L59 (137.8349, 16.4831) -> (136.4025, 12.5704) projected
  line L60 (136.4025, 12.5704) -> (133.9025, 12.5705) projected
  line L61 (133.9025, 12.5705) -> (135.3349, 16.4832) projected
  line L62 (145.3349, 16.4827) -> (147.8349, 16.4825) projected
  line L63 (147.8349, 16.4825) -> (146.4025, 12.5699) projected
  line L64 (146.4025, 12.5699) -> (143.9025, 12.57) projected
  line L65 (143.9025, 12.57) -> (145.3349, 16.4827) projected
  line L66 (155.3349, 16.4821) -> (157.8349, 16.482) projected
  line L67 (157.8349, 16.482) -> (156.4025, 12.5693) projected
  line L68 (156.4025, 12.5693) -> (153.9025, 12.5695) projected
  line L69 (153.9025, 12.5695) -> (155.3349, 16.4821) projected
  line L70 (165.3349, 16.4816) -> (167.8349, 16.4815) projected
  line L71 (167.8349, 16.4815) -> (166.4025, 12.5688) projected
  line L72 (166.4025, 12.5688) -> (163.9025, 12.5689) projected
  line L73 (163.9025, 12.5689) -> (165.3349, 16.4816) projected
  line L74 (175.3349, 16.4811) -> (177.8349, 16.4809) projected
  line L75 (177.8349, 16.4809) -> (176.4025, 12.5683) projected
  line L76 (176.4025, 12.5683) -> (173.9025, 12.5684) projected
  line L77 (173.9025, 12.5684) -> (175.3349, 16.4811) projected
  line L78 (170.3349, 16.4813) -> (172.8349, 16.4812) projected
  line L79 (172.8349, 16.4812) -> (171.4025, 12.5685) projected
  line L80 (171.4025, 12.5685) -> (168.9025, 12.5687) projected
  line L81 (168.9025, 12.5687) -> (170.3349, 16.4813) projected
  line L82 (160.3349, 16.4819) -> (162.8349, 16.4817) projected
  line L83 (162.8349, 16.4817) -> (161.4025, 12.5691) projected
  line L84 (161.4025, 12.5691) -> (158.9025, 12.5692) projected
  line L85 (158.9025, 12.5692) -> (160.3349, 16.4819) projected
  line L86 (150.3349, 16.4824) -> (152.8349, 16.4823) projected
  line L87 (152.8349, 16.4823) -> (151.4025, 12.5696) projected
  line L88 (151.4025, 12.5696) -> (148.9025, 12.5697) projected
  line L89 (148.9025, 12.5697) -> (150.3349, 16.4824) projected
  line L90 (140.3349, 16.4829) -> (142.8349, 16.4828) projected
  line L91 (142.8349, 16.4828) -> (141.4025, 12.5701) projected
  line L92 (141.4025, 12.5701) -> (138.9025, 12.5703) projected
  line L93 (138.9025, 12.5703) -> (140.3349, 16.4829) projected
  line L94 (130.3349, 16.4835) -> (132.8349, 16.4833) projected
  line L95 (132.8349, 16.4833) -> (131.4025, 12.5707) projected
  line L96 (131.4025, 12.5707) -> (128.9025, 12.5708) projected
  line L97 (128.9025, 12.5708) -> (130.3349, 16.4835) projected
  line L98 (120.3349, 16.484) -> (122.8349, 16.4839) projected
  line L99 (122.8349, 16.4839) -> (121.4025, 12.5712) projected
  line L100 (121.4025, 12.5712) -> (118.9025, 12.5713) projected
  line L101 (118.9025, 12.5713) -> (120.3349, 16.484) projected
  line L102 (110.3349, 16.4845) -> (112.8349, 16.4844) projected
  line L103 (112.8349, 16.4844) -> (111.4025, 12.5717) projected
  line L104 (111.4025, 12.5717) -> (108.9025, 12.5719) projected
  line L105 (108.9025, 12.5719) -> (110.3349, 16.4845) projected
  line L106 (100.3352, 16.4851) -> (102.8352, 16.4849) projected
  line L107 (102.8352, 16.4849) -> (101.4027, 12.5723) projected
  line L108 (101.4027, 12.5723) -> (98.9027, 12.5724) projected
  line L109 (98.9027, 12.5724) -> (100.3352, 16.4851) projected
  line L110 (177.8342, 2.822) -> (174.2947, -6.8462) projected
  line L111 (174.2947, -6.8462) -> (171.7947, -6.846) projected
  line L112 (171.7947, -6.846) -> (177.8346, 9.6518) projected
  line L113 (177.8346, 9.6518) -> (177.8342, 2.822) projected
  line L114 (110.7291, 10.7322) -> (104.2949, -6.8424) projected
  line L115 (104.2949, -6.8424) -> (101.7949, -6.8423) projected
  line L116 (101.7949, -6.8423) -> (108.2291, 10.7324) projected
  line L117 (108.2291, 10.7324) -> (110.7291, 10.7322) projected
  line L118 (120.7291, 10.7317) -> (114.2949, -6.843) projected
  line L119 (114.2949, -6.843) -> (111.7949, -6.8428) projected
  line L120 (111.7949, -6.8428) -> (118.2291, 10.7318) projected
  line L121 (118.2291, 10.7318) -> (120.7291, 10.7317) projected
  line L122 (130.7291, 10.7312) -> (124.2949, -6.8435) projected
  line L123 (124.2949, -6.8435) -> (121.7949, -6.8434) projected
  line L124 (121.7949, -6.8434) -> (128.2291, 10.7313) projected
  line L125 (128.2291, 10.7313) -> (130.7291, 10.7312) projected
  line L126 (140.7291, 10.7306) -> (134.2949, -6.844) projected
  line L127 (134.2949, -6.844) -> (131.7949, -6.8439) projected
  line L128 (131.7949, -6.8439) -> (138.2291, 10.7308) projected
  line L129 (138.2291, 10.7308) -> (140.7291, 10.7306) projected
  line L130 (150.7291, 10.7301) -> (144.2949, -6.8446) projected
  line L131 (144.2949, -6.8446) -> (141.7949, -6.8444) projected
  line L132 (141.7949, -6.8444) -> (148.2291, 10.7302) projected
  line L133 (148.2291, 10.7302) -> (150.7291, 10.7301) projected
  line L134 (160.7291, 10.7296) -> (154.2949, -6.8451) projected
  line L135 (154.2949, -6.8451) -> (151.7949, -6.845) projected
  line L136 (151.7949, -6.845) -> (158.2291, 10.7297) projected
  line L137 (158.2291, 10.7297) -> (160.7291, 10.7296) projected
  line L138 (170.7291, 10.729) -> (164.2949, -6.8456) projected
  line L139 (164.2949, -6.8456) -> (161.7949, -6.8455) projected
  line L140 (161.7949, -6.8455) -> (168.2291, 10.7292) projected
  line L141 (168.2291, 10.7292) -> (170.7291, 10.729) projected
  line L142 (42.8372, 16.4881) -> (97.8349, 16.4852) projected
  line L143 (97.8349, 16.4852) -> (96.4025, 12.5725) projected
  line L144 (96.4025, 12.5725) -> (41.4047, 12.5755) projected
  line L145 (41.4047, 12.5755) -> (42.8372, 16.4881) projected
  line L146 (41.4046, 10.7359) -> (93.6046, 10.7332) projected
  line L147 (93.6046, 10.7332) -> (93.6037, -6.9463) projected
  line L148 (93.6037, -6.9463) -> (41.4037, -6.9435) projected
  line L149 (41.4037, -6.9435) -> (41.4046, 10.7359) projected
  line L150 (-194.9318, 78.1502) -> (-194.931, 92.071) projected
  line L151 (-194.931, 92.071) -> (-180.931, 92.0702) projected
  line L152 (-180.931, 92.0702) -> (-180.9318, 78.1494) projected
  line L153 (-180.9318, 78.1494) -> (-194.9318, 78.1502) projected
  line L154 (-175.9318, 78.1491) -> (-175.931, 92.07) projected
  line L155 (-175.931, 92.07) -> (-161.931, 92.0692) projected
  line L156 (-161.931, 92.0692) -> (-161.9318, 78.1484) projected
  line L157 (-161.9318, 78.1484) -> (-175.9318, 78.1491) projected
  line L158 (-156.9318, 78.1481) -> (-156.931, 92.0689) projected
  line L159 (-156.931, 92.0689) -> (-142.931, 92.0682) projected
  line L160 (-142.931, 92.0682) -> (-142.9318, 78.1474) projected
  line L161 (-142.9318, 78.1474) -> (-156.9318, 78.1481) projected
  line L162 (-137.9318, 78.1471) -> (-137.931, 92.0679) projected
  line L163 (-137.931, 92.0679) -> (-123.931, 92.0672) projected
  line L164 (-123.931, 92.0672) -> (-123.9318, 78.1464) projected
  line L165 (-123.9318, 78.1464) -> (-137.9318, 78.1471) projected
  line L166 (-118.9318, 78.1461) -> (-118.931, 92.0669) projected
  line L167 (-118.931, 92.0669) -> (-104.931, 92.0662) projected
  line L168 (-104.931, 92.0662) -> (-104.9318, 78.1453) projected
  line L169 (-104.9318, 78.1453) -> (-118.9318, 78.1461) projected
  line L170 (-99.9318, 78.1451) -> (-99.931, 92.0659) projected
  line L171 (-99.931, 92.0659) -> (-85.931, 92.0651) projected
  line L172 (-85.931, 92.0651) -> (-85.9318, 78.1443) projected
  line L173 (-85.9318, 78.1443) -> (-99.9318, 78.1451) projected
  line L174 (-80.9318, 78.1441) -> (-80.931, 92.0649) projected
  line L175 (-80.931, 92.0649) -> (-66.931, 92.0641) projected
  line L176 (-66.931, 92.0641) -> (-66.9318, 78.1433) projected
  line L177 (-66.9318, 78.1433) -> (-80.9318, 78.1441) projected
  line L178 (-61.9318, 78.1431) -> (-61.931, 92.0639) projected
  line L179 (-61.931, 92.0639) -> (-47.931, 92.0631) projected
  line L180 (-47.931, 92.0631) -> (-47.9318, 78.1423) projected
  line L181 (-47.9318, 78.1423) -> (-61.9318, 78.1431) projected
  line L182 (-42.9318, 78.142) -> (-42.931, 92.0629) projected
  line L183 (-42.931, 92.0629) -> (-28.931, 92.0621) projected
  line L184 (-28.931, 92.0621) -> (-28.9318, 78.1413) projected
  line L185 (-28.9318, 78.1413) -> (-42.9318, 78.142) projected
  line L186 (-190.4328, 59.2574) -> (-204.4328, 59.2581) projected
  line L187 (-204.4328, 59.2581) -> (-204.432, 73.1789) projected
  line L188 (-204.432, 73.1789) -> (-190.432, 73.1782) projected
  line L189 (-190.432, 73.1782) -> (-190.4328, 59.2574) projected
  line L190 (-171.4328, 59.2564) -> (-185.4328, 59.2571) projected
  line L191 (-185.4328, 59.2571) -> (-185.432, 73.1779) projected
  line L192 (-185.432, 73.1779) -> (-171.432, 73.1772) projected
  line L193 (-171.432, 73.1772) -> (-171.4328, 59.2564) projected
  line L194 (-152.4328, 59.2554) -> (-166.4328, 59.2561) projected
  line L195 (-166.4328, 59.2561) -> (-166.432, 73.1769) projected
  line L196 (-166.432, 73.1769) -> (-152.432, 73.1762) projected
  line L197 (-152.432, 73.1762) -> (-152.4328, 59.2554) projected
  line L198 (-133.4328, 59.2543) -> (-147.4328, 59.2551) projected
  line L199 (-147.4328, 59.2551) -> (-147.432, 73.1759) projected
  line L200 (-147.432, 73.1759) -> (-133.432, 73.1752) projected
  line L201 (-133.432, 73.1752) -> (-133.4328, 59.2543) projected
  line L202 (-114.4328, 59.2533) -> (-128.4328, 59.2541) projected
  line L203 (-128.4328, 59.2541) -> (-128.432, 73.1749) projected
  line L204 (-128.432, 73.1749) -> (-114.432, 73.1741) projected
  line L205 (-114.432, 73.1741) -> (-114.4328, 59.2533) projected
  line L206 (-95.4328, 59.2523) -> (-109.4328, 59.2531) projected
  line L207 (-109.4328, 59.2531) -> (-109.432, 73.1739) projected
  line L208 (-109.432, 73.1739) -> (-95.432, 73.1731) projected
  line L209 (-95.432, 73.1731) -> (-95.4328, 59.2523) projected
  line L210 (-76.4328, 59.2513) -> (-90.4328, 59.252) projected
  line L211 (-90.4328, 59.252) -> (-90.432, 73.1729) projected
  line L212 (-90.432, 73.1729) -> (-76.432, 73.1721) projected
  line L213 (-76.432, 73.1721) -> (-76.4328, 59.2513) projected
  line L214 (-57.4328, 59.2503) -> (-71.4328, 59.251) projected
  line L215 (-71.4328, 59.251) -> (-71.432, 73.1718) projected
  line L216 (-71.432, 73.1718) -> (-57.432, 73.1711) projected
  line L217 (-57.432, 73.1711) -> (-57.4328, 59.2503) projected
  line L218 (-38.4328, 59.2493) -> (-52.4328, 59.25) projected
  line L219 (-52.4328, 59.25) -> (-52.432, 73.1708) projected
  line L220 (-52.432, 73.1708) -> (-38.432, 73.1701) projected
  line L221 (-38.432, 73.1701) -> (-38.4328, 59.2493) projected
  line L222 (-19.4328, 59.2483) -> (-33.4328, 59.249) projected
  line L223 (-33.4328, 59.249) -> (-33.432, 73.1698) projected
  line L224 (-33.432, 73.1698) -> (-19.432, 73.1691) projected
  line L225 (-19.432, 73.1691) -> (-19.4328, 59.2483) projected
  line L226 (-218.6838, 40.3664) -> (-218.683, 54.2872) projected
  line L227 (-218.683, 54.2872) -> (-204.683, 54.2864) projected
  line L228 (-204.683, 54.2864) -> (-204.6838, 40.3656) projected
  line L229 (-204.6838, 40.3656) -> (-218.6838, 40.3664) projected
  line L230 (-199.6838, 40.3653) -> (-199.683, 54.2862) projected
  line L231 (-199.683, 54.2862) -> (-185.683, 54.2854) projected
  line L232 (-185.683, 54.2854) -> (-185.6838, 40.3646) projected
  line L233 (-185.6838, 40.3646) -> (-199.6838, 40.3653) projected
  line L234 (-180.6838, 40.3643) -> (-180.683, 54.2851) projected
  line L235 (-180.683, 54.2851) -> (-166.683, 54.2844) projected
  line L236 (-166.683, 54.2844) -> (-166.6838, 40.3636) projected
  line L237 (-166.6838, 40.3636) -> (-180.6838, 40.3643) projected
  line L238 (-161.6838, 40.3633) -> (-161.683, 54.2841) projected
  line L239 (-161.683, 54.2841) -> (-147.683, 54.2834) projected
  line L240 (-147.683, 54.2834) -> (-147.6838, 40.3626) projected
  line L241 (-147.6838, 40.3626) -> (-161.6838, 40.3633) projected
  line L242 (-142.6838, 40.3623) -> (-142.683, 54.2831) projected
  line L243 (-142.683, 54.2831) -> (-128.683, 54.2824) projected
  line L244 (-128.683, 54.2824) -> (-128.6838, 40.3616) projected
  line L245 (-128.6838, 40.3616) -> (-142.6838, 40.3623) projected
  line L246 (-123.6838, 40.3613) -> (-123.683, 54.2821) projected
  line L247 (-123.683, 54.2821) -> (-109.683, 54.2814) projected
  line L248 (-109.683, 54.2814) -> (-109.6838, 40.3605) projected
  line L249 (-109.6838, 40.3605) -> (-123.6838, 40.3613) projected
  line L250 (-104.6838, 40.3603) -> (-104.683, 54.2811) projected
  line L251 (-104.683, 54.2811) -> (-90.683, 54.2803) projected
  line L252 (-90.683, 54.2803) -> (-90.6838, 40.3595) projected
  line L253 (-90.6838, 40.3595) -> (-104.6838, 40.3603) projected
  line L254 (-85.6838, 40.3593) -> (-85.683, 54.2801) projected
  line L255 (-85.683, 54.2801) -> (-71.683, 54.2793) projected
  line L256 (-71.683, 54.2793) -> (-71.6838, 40.3585) projected
  line L257 (-71.6838, 40.3585) -> (-85.6838, 40.3593) projected
  line L258 (-66.6838, 40.3582) -> (-66.683, 54.2791) projected
  line L259 (-66.683, 54.2791) -> (-52.683, 54.2783) projected
  line L260 (-52.683, 54.2783) -> (-52.6838, 40.3575) projected
  line L261 (-52.6838, 40.3575) -> (-66.6838, 40.3582) projected
  line L262 (-47.6838, 40.3572) -> (-47.683, 54.278) projected
  line L263 (-47.683, 54.278) -> (-33.683, 54.2773) projected
  line L264 (-33.683, 54.2773) -> (-33.6838, 40.3565) projected
  line L265 (-33.6838, 40.3565) -> (-47.6838, 40.3572) projected
  line L266 (-28.6838, 40.3562) -> (-28.683, 54.277) projected
  line L267 (-28.683, 54.277) -> (-14.683, 54.2763) projected
  line L268 (-14.683, 54.2763) -> (-14.6838, 40.3555) projected
  line L269 (-14.6838, 40.3555) -> (-28.6838, 40.3562) projected
  line L270 (-23.9318, 78.141) -> (-23.931, 92.0618) projected
  line L271 (-23.931, 92.0618) -> (-9.931, 92.0611) projected
  line L272 (-9.931, 92.0611) -> (-9.9318, 78.1403) projected
  line L273 (-9.9318, 78.1403) -> (-23.9318, 78.141) projected
  line L274 (-14.4328, 59.248) -> (-14.432, 73.1688) projected
  line L275 (-14.432, 73.1688) -> (-0.432, 73.1681) projected
  line L276 (-0.432, 73.1681) -> (-0.4328, 59.2472) projected
  line L277 (-0.4328, 59.2472) -> (-14.4328, 59.248) projected
  line L278 (-9.6838, 40.3552) -> (-9.683, 54.276) projected
  line L279 (-9.683, 54.276) -> (4.317, 54.2753) projected
  line L280 (4.317, 54.2753) -> (4.3162, 40.3545) projected
  line L281 (4.3162, 40.3545) -> (-9.6838, 40.3552) projected
  line L282 (-237.6848, 21.4748) -> (-237.6841, 35.3957) projected
  line L283 (-237.6841, 35.3957) -> (-223.6841, 35.3949) projected
  line L284 (-223.6841, 35.3949) -> (-223.6848, 21.4741) projected
  line L285 (-223.6848, 21.4741) -> (-237.6848, 21.4748) projected
  line L286 (-242.4338, 40.3676) -> (-242.433, 54.2884) projected
  line L287 (-242.433, 54.2884) -> (-228.433, 54.2877) projected
  line L288 (-228.433, 54.2877) -> (-228.4338, 40.3669) projected
  line L289 (-228.4338, 40.3669) -> (-242.4338, 40.3676) projected
  line L290 (-235.3078, 59.2598) -> (-235.307, 73.1806) projected
  line L291 (-235.307, 73.1806) -> (-221.307, 73.1798) projected
  line L292 (-221.307, 73.1798) -> (-221.3078, 59.259) projected
  line L293 (-221.3078, 59.259) -> (-235.3078, 59.2598) projected
  line L294 (-230.5568, 78.1521) -> (-230.556, 92.0729) projected
  line L295 (-230.556, 92.0729) -> (-216.556, 92.0721) projected
  line L296 (-216.556, 92.0721) -> (-216.5568, 78.1513) projected
  line L297 (-216.5568, 78.1513) -> (-230.5568, 78.1521) projected
  line L298 (-244.8058, 97.0454) -> (-244.805, 110.9662) projected
  line L299 (-244.805, 110.9662) -> (-230.805, 110.9654) projected
  line L300 (-230.805, 110.9654) -> (-230.8058, 97.0446) projected
  line L301 (-230.8058, 97.0446) -> (-244.8058, 97.0454) projected
  line L302 (-221.0558, 97.0441) -> (-221.055, 110.9649) projected
  line L303 (-221.055, 110.9649) -> (-207.055, 110.9641) projected
  line L304 (-207.055, 110.9641) -> (-207.0558, 97.0433) projected
  line L305 (-207.0558, 97.0433) -> (-221.0558, 97.0441) projected
  line L306 (-197.3058, 97.0428) -> (-197.305, 110.9636) projected
  line L307 (-197.305, 110.9636) -> (-183.305, 110.9629) projected
  line L308 (-183.305, 110.9629) -> (-183.3058, 97.0421) projected
  line L309 (-183.3058, 97.0421) -> (-197.3058, 97.0428) projected
  line L310 (-114.1808, 97.0384) -> (-114.18, 110.9592) projected
  line L311 (-114.18, 110.9592) -> (-100.18, 110.9584) projected
  line L312 (-100.18, 110.9584) -> (-100.1808, 97.0376) projected